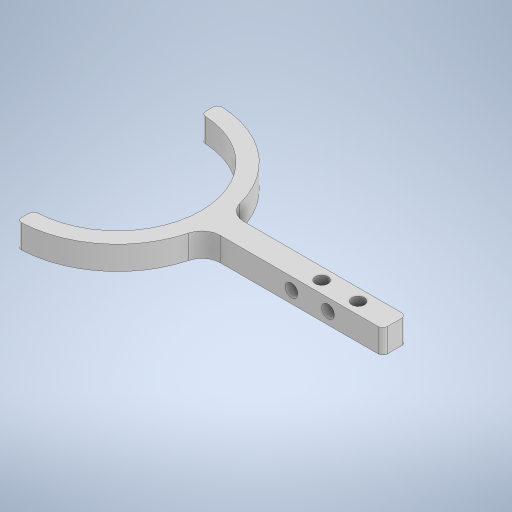
# Autodesk Inventor part: stojak
Saved by Autodesk Inventor 2024.2 (Build 282272000, 272)
## iProperties
Created: 2024-06-19
Part Number: stojak
Material: Ogólny
Document SubType Name: Modeling
Designer: Konrad
Density: 1 g/cm^3
Appearance: Domyślna
Author: Konrad
Autodesk Inventor part; units mm, degrees
ref_plane "YZ Plane" through (0, 0, 0) normal (1, 0, 0) x (0, 1, 0)
ref_plane "XZ Plane" through (0, 0, 0) normal (0, 1, 0) x (-1, 0, 0)
ref_plane "XY Plane" through (0, 0, 0) normal (0, 0, 1) x (1, 0, 0)
sketch "Szkic1" plane through (0, 0, 0) normal (0, 1, 0) x (-1, 0, 0)
  circle A0 centre (0, 0) radius 23 construction
  arc A1 (0, 23) -> (0, -23) centre (0, 0) ccw
  line L0 (0, 23) -> (0, 27.5)
  line L1 (0, -23) -> (0, -27.5)
  line L2 (0, -38.5) -> (0, 38.5) projected
  arc A2 (0, 27.5) -> (0, -27.5) centre (0, 0) ccw
  line L3 (-76, 3.25) -> (-27.3073, 3.25)
  line L4 (-27.3073, 3.25) -> (-27.3073, -3.25) construction
  line L5 (-27.3073, -3.25) -> (-76, -3.25)
  line L6 (-76, -3.25) -> (-76, 3.25)
  line L7 (42.8, 0) -> (-95.8, 0) projected
  circle A3 centre (-66, 0) radius 1.75
  circle A4 centre (-56, 0) radius 1.75
  point P0 (-27.5, 0)
  point P1 (-23, 0)
  dimension "d0" = 46
  dimension "d1" = 4.5
  dimension "d2" = 4.5
  dimension "d3" = 6.5
  dimension "d4" = 76
  dimension "d5" = 3.5
  dimension "d6" = 10
  dimension "d7" = 10
  constraints: 12 end point, 9 point on circle, 5 centre point, 4 point on line, 2 parallel, 2 vertical, 1 coincident, 1 collinear, 1 concentric, 1 equal radius, 1 horizontal, 1 perpendicular, 1 other
  measures "d0" diameter of A0
  measures "d1" distance of L1.start L1.end
  measures "d2" distance of point (-27.5, 0) point (-23, 0)
  measures "d3" distance of L5.end L3.start
  measures "d4" distance from line of L6 point (0, 0)
  measures "d5" diameter of A3
  measures "d6" distance from line of L6 A3.centre
  measures "d7" distance of A4.centre A3.centre
extrude "Wyciągnięcie proste1" add sketch "Szkic1" along normal blind 6.5 contours A1 L7 A2 L0 | A1 L1 A2 L7 | L7 A4 A3 L6 L3 A2 | A2 L5 L6 L7 A3 A4
sketch "Szkic2" plane through (76, 0, -3.25) normal (0, 0, -1) x (-1, 0, 0)
  line L0 (0, 0) -> (48.6927, 0) projected
  line L1 (48.6927, 0) -> (48.6927, 6.5) projected
  line L2 (0, 6.5) -> (48.6927, 6.5) projected
  line L3 (0, 0) -> (0, 6.5) projected
  line L4 (48.6927, 0) -> (48.6927, 6.5) projected
  line L5 (48.6927, 3.25) -> (0, 3.25) construction
  circle A0 centre (15, 3.25) radius 1.75
  circle A1 centre (25, 3.25) radius 1.75
  point P0 (76, 0)
  dimension "d10" = 3.5
  dimension "d11" = 3.5
  dimension "d12" = 15
  dimension "d13" = 10
  constraints: 2 centre point, 2 end point, 2 midpoint, 2 point on line
  measures "d10" diameter of A0
  measures "d11" diameter of A1
  measures "d12" distance from line of L3 A0.centre
  measures "d13" distance of A0.centre A1.centre
extrude "Wyciągnięcie proste2" cut sketch "Szkic2" against normal up to surface (6.5 mm away) contours A0 | A1
fillet "Zaokrąglenie1" radius 5 2 edges at (27.3073, 3.25, 3.25) (27.3073, 3.25, -3.25)
fillet "Zaokrąglenie2" radius 1.2 6 edges at (0, 3.25, 27.5) (0, 3.25, 23) (0, 3.25, -23) (0, 3.25, -27.5) (76, 3.25, 3.25) (76, 3.25, -3.25)
equation "\"d2\" = d1"
equation "\"d8\" = d3"
equation "\"d14\" = d3"
